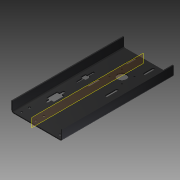
# Autodesk Inventor part: simple_upright
Saved by Autodesk Inventor 2014 (Build 180170000, 170)
## iProperties
Created: 2013-07-18
Part Number: simple_upright
Material: Steel, Mild
Document SubType Name: Sheet Metal
Designer: Edward
Density: 7.86 g/cm^3
Sheet Metal Rule: Default
Appearance: Lacquer - Black
Flat Pattern Width: 16.6565 cm
Flat Pattern Length: 27.5 cm
Flat Pattern Area: 458.052 cm^2
Sheet Metal Width: 166.565 mm
Sheet Metal Length: 275.000 mm
Sheet Metal Area: 45805.249 mm^2
Author: Edward
Autodesk Inventor part; units mm, degrees
ref_plane "YZ Plane" through (0, 0, 0) normal (1, 0, 0) x (0, 1, 0)
ref_plane "XZ Plane" through (0, 0, 0) normal (0, 1, 0) x (-1, 0, 0)
ref_plane "XY Plane" through (0, 0, 0) normal (0, 0, 1) x (1, 0, 0)
sketch "Sketch1" plane through (0, 0, 0) normal (0, 0, 1) x (1, 0, 0)
  line L0 (-50, 125) -> (75, 125)
  line L1 (75, 125) -> (75, -150)
  line L2 (75, -150) -> (-50, -150)
  line L3 (-50, -150) -> (-50, 125)
  point P0 (0, 0)
  dimension "d0" = 125
  dimension "d1" = 275
  dimension "d2" = 50
  dimension "d3" = 125
  measures "d0" distance of L1.end L2.end
  measures "d1" distance of L0.end L1.end
  measures "d2" distance from line of point (0, 0) L3
  measures "d3" distance from line of L0 point (0, 0)
extrude "Plate1" add sketch "Sketch1" along normal blind 2.6568
sketch "Sketch2" plane through (72.3432, 125, 0) normal (1, 0, 0) x (0, 1, 0)
  line L0 (-275, 0) -> (0, 0)
  line L1 (0, 0) -> (0, 25.4)
  line L2 (0, 25.4) -> (-275, 25.4)
  line L3 (-275, 25.4) -> (-275, 0)
  constraints: 6 end point, 1 horizontal, 1 perpendicular, 1 vertical
edge flange "Flange1" height 25.4 angle 90 thickness 2.6568 bend radius 2.6568 thickness toward (1, 0, 0) relief straight relief width 2.6568 relief depth 1.3284 corner gap 2.6568 corner form 0 edges at (75, -12.5, 2.6568) (-50, -12.5, 2.6568) wall of the first edge with corners at (72.3432, -150, 0) (72.3432, 125, 0) (72.3432, 125, 25.4) (72.3432, -150, 25.4)
bend "Bend1"
corner "Corner1"
sketch "Sketch3" plane through (0, 0, 2.6568) normal (0, 0, 1) x (1, 0, 0)
  line L0 (-44.6863, 125) -> (-44.6863, -150) projected
  line L1 (-44.6863, 125) -> (69.6863, 125) projected
  circle A0 centre (12.5, 60) radius 11.25
  circle A1 centre (-3, 75.5) radius 1.75
  circle A2 centre (28, 75.5) radius 1.75
  circle A3 centre (-3, 44.5) radius 1.75
  circle A4 centre (28, 44.5) radius 1.75
  line L2 (69.6863, -150) -> (69.6863, 125) projected
  point P0 (0, 0)
  dimension "d15" = 22.5
  dimension "d16" = 65
  dimension "d17" = 3.5
  dimension "d18" = 15.5
  dimension "d19" = 15.5
  dimension "d22" = 31
  dimension "d25" = 31
  dimension "d30" = 57.1863
  constraints: 5 centre point, 1 horizontal, 1 vertical, 6 other
  measures "d15" diameter of A0
  measures "d16" distance from line of L1 A0.centre
  measures "d17" diameter of A1
  measures "d18" horizontal distance of A1.centre A0.centre
  measures "d19" horizontal distance of A0.centre A1.centre
  measures "d22" distance of A1.centre A2.centre
  measures "d25" distance of A1.centre A3.centre
  measures "d30" distance from line of L2 A0.centre
extrude "Extrusion1" cut sketch "Sketch3" against normal through all
sketch "Sketch4" plane through (0, 0, 2.6568) normal (0, 0, 1) x (1, 0, 0)
  line L0 (-44.6863, 125) -> (-44.6863, -150) projected
  line L1 (69.6863, -150) -> (69.6863, 125) projected
  line L2 (-44.6863, 125) -> (69.6863, 125) projected
  line L3 (34.85, 115) -> (34.85, 94) construction
  line L4 (32.1, 115) -> (32.1, 94)
  line L5 (37.6, 94) -> (37.6, 115)
  arc A0 (37.6, 115) -> (32.1, 115) centre (34.85, 115) ccw
  arc A1 (32.1, 94) -> (37.6, 94) centre (34.85, 94) ccw
  line L6 (34.85, 115) -> (55.85, 115) construction
  line L7 (34.85, 25) -> (34.85, 0) construction
  line L8 (32.1, 25) -> (32.1, 0)
  line L9 (37.6, 0) -> (37.6, 25)
  arc A2 (37.6, 25) -> (32.1, 25) centre (34.85, 25) ccw
  arc A3 (32.1, 0) -> (37.6, 0) centre (34.85, 0) ccw
  line L10 (34.85, 25) -> (59.85, 25) construction
  point P0 (0, 0)
  point P1 (34.85, 104.5)
  point P2 (34.85, 12.5)
  dimension "d31" = 21
  dimension "d32" = 90
  dimension "d33" = 5.5
  dimension "d34" = 10
  dimension "d35" = 34.8363
  dimension "d36" = 25
  dimension "d37" = 90
  dimension "d38" = 5.5
  dimension "d39" = 100
  dimension "d40" = 34.8363
  constraints: 20 end point, 8 point on circle, 8 tangent, 4 centre point, 4 parallel, 2 horizontal, 2 midpoint, 2 perpendicular
  measures "d31" distance of L3.start L3.end
  measures "d32" angle of L3 L6
  measures "d33" diameter of A1
  measures "d34" distance from line of L2 L3.start
  measures "d35" distance from line of L1 L3.start
  measures "d36" distance of L7.start L7.end
  measures "d37" angle of L7 L10
  measures "d38" diameter of A3
  measures "d39" distance from line of L2 L7.start
  measures "d40" distance from line of L1 L7.start
extrude "Extrusion2" cut sketch "Sketch4" against normal through all
ref_plane "Work Plane1" through (12.5, -150, 25.4) normal (1, 0, 0) x (0, 0, -1)
mirror "Mirror1" about plane through (12.5, -150, 25.4) normal (1, 0, 0) of "Extrusion2"
sketch "Sketch5" plane through (0, 0, 2.6568) normal (0, 0, 1) x (1, 0, 0)
  line L0 (-18.3432, -55) -> (-18.3432, -75) projected
  line L1 (-34.3432, -73) -> (-34.3432, -57) projected
  line L2 (-20.3432, -53) -> (-30.3432, -53) projected
  line L3 (-20.3432, -77) -> (-30.3432, -77) projected
  circle A0 centre (-26.3432, -45) radius 2.7 projected
  circle A1 centre (-26.3432, -85) radius 2.7 projected
  line L4 (-17.3432, -52) -> (-17.3432, -78)
  line L5 (-35.3432, -78) -> (-35.3432, -52)
  arc A2 (-23.3432, -45) -> (-29.3432, -45) centre (-26.3432, -45) ccw
  arc A3 (-29.3432, -85) -> (-23.3432, -85) centre (-26.3432, -85) ccw
  line L6 (-29.3432, -45) -> (-29.3432, -52)
  line L7 (-23.3432, -45) -> (-23.3432, -52)
  line L8 (-35.3432, -52) -> (-29.3432, -52)
  line L9 (-23.3432, -52) -> (-17.3432, -52)
  line L10 (-29.3432, -85) -> (-29.3432, -78)
  line L11 (-23.3432, -85) -> (-23.3432, -78)
  line L12 (-17.3432, -78) -> (-23.3432, -78)
  line L13 (-29.3432, -78) -> (-35.3432, -78)
  point P0 (0, 0)
  dimension "d44" = 1
  dimension "d45" = 1
  dimension "d48" = 6
  dimension "d49" = 6
  constraints: 20 end point, 9 perpendicular, 5 parallel, 4 point on circle, 4 tangent, 2 centre point, 2 coincident, 2 horizontal
  measures "d44" distance between parallel lines of L4 L0
  measures "d45" distance between parallel lines of L1 L5
  measures "d48" diameter of A2
  measures "d49" diameter of A3
extrude "ac_power" cut sketch "Sketch5" against normal through all contours A0 | A1 | L4 L12 L11 A3 L10 L13 L5 L8 L6 A2 L7 L9
sketch "Sketch6" plane through (0, 0, 2.6568) normal (0, 0, 1) x (1, 0, 0)
  line L0 (-25.1081, 20.3256) -> (-25.1081, 7.8256)
  line L1 (-37.6081, 7.8256) -> (-37.6081, 20.3256)
  arc A0 (-29.3581, 33.8256) -> (-33.3581, 33.8256) centre (-31.3581, 33.8256) ccw
  arc A1 (-33.3581, -5.6744) -> (-29.3581, -5.6744) centre (-31.3581, -5.6744) ccw
  line L2 (-33.3581, 33.8256) -> (-33.3581, 20.3256)
  line L3 (-29.3581, 33.8256) -> (-29.3581, 20.3256)
  line L4 (-33.3581, -5.6744) -> (-33.3581, 7.8256)
  line L5 (-29.3581, -5.6744) -> (-29.3581, 7.8256)
  line L6 (-25.1081, 7.8256) -> (-29.3581, 7.8256)
  line L7 (-33.3581, 7.8256) -> (-37.6081, 7.8256)
  line L8 (-37.6081, 20.3256) -> (-33.3581, 20.3256)
  line L9 (-29.3581, 20.3256) -> (-25.1081, 20.3256)
  point P0 (0, 0)
  dimension "d52" = 12.5
  dimension "d53" = 12.5
  dimension "d56" = 4
  dimension "d58" = 4
  constraints: 20 end point, 10 perpendicular, 5 parallel, 4 point on circle, 4 tangent, 2 centre point, 2 horizontal
  measures "d52" distance of L0.end L1.start
  measures "d53" distance of L0.start L0.end
  measures "d56" diameter of A0
  measures "d58" diameter of A1
extrude "usb_panel" cut sketch "Sketch6" against normal through all
sketch "Sketch7" plane through (0, 0, 2.6568) normal (0, 0, 1) x (1, 0, 0)
  line L0 (69.6863, -150) -> (-44.6863, -150) projected
  line L1 (69.6863, -150) -> (69.6863, 125) projected
  circle A0 centre (-35.3432, -140) radius 2.75
  circle A1 centre (0, -140) radius 2.75
  circle A2 centre (59.6863, -140) radius 2.75
  point P0 (0, 0)
  dimension "d62" = 5.5
  dimension "d63" = 10
  dimension "d64" = 5.5
  dimension "d65" = 5.5
  dimension "d66" = 10
  dimension "d67" = 10
  dimension "d68" = 10
  constraints: 3 centre point
  measures "d62" diameter of A0
  measures "d63" distance from line of L0 A0.centre
  measures "d64" diameter of A1
  measures "d65" diameter of A2
  measures "d66" distance from line of L1 A2.centre
  measures "d67" distance from line of L0 A1.centre
  measures "d68" distance from line of L0 A2.centre
extrude "Extrusion5" cut sketch "Sketch7" against normal through all
pattern_linear "Rectangular Pattern1" count 2 spacing 20 along (0, 1, 0) of "Extrusion5"
equation "\"d40\" = d35"
equation "\"d67\" = d63"
equation "\"d68\" = d63"
equation "\"d5\" = BendReliefWidth"
equation "\"d6\" = BendReliefDepth"
equation "\"d7\" = MinimumRemnant"
equation "\"d8\" = BendRadius"
equation "\"d11\" = BendRadius"
equation "\"d12\" = CornerReliefSize"
equation "\"d13\" = GapSize"
equation "\"d14\" = JacobiRadiusSize"
equation "\"BendRadius\" = Thickness"
equation "\"BendReliefWidth\" = Thickness"
equation "\"BendReliefDepth\" = 0.5 * Thickness"
equation "\"CornerReliefSize\" = 4 * Thickness"
equation "\"MinimumRemnant\" = 2 * Thickness"
equation "\"TransitionRadius\" = BendRadius"
equation "\"JacobiRadiusSize\" = Thickness"
equation "\"GapSize\" = Thickness"
equation "\"d4\" = BendRadius"
equation "\"Thickness\" = 2.65684"
body "Solid1"
